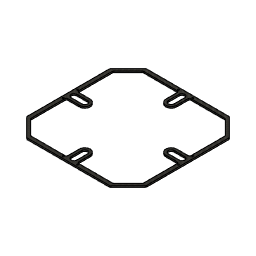
CarbonFiberBoardDown (Autodesk Fusion 360 design; units mm, degrees)
Autodesk Fusion 360 part; units mm, degrees
sketch "草图1" plane through (0, 0, 0) normal (0, 0, 1) x (1, 0, 0)
  line L0 (7.5, 60) -> (7.5, 75)
  circle A0 centre (-42.5, 42.5) radius 32.5 construction
  arc A1 (-7.5, 60) -> (7.5, 60) centre (0, 60) ccw
  circle A2 centre (42.5, 42.5) radius 32.5 construction
  circle A3 centre (-10, 80) radius 1.05
  line L1 (-7.5, 75) -> (-7.5, 60)
  line L2 (57.8614, 83) -> (0, 83)
  line L3 (0, 60) -> (0, 75) construction
  circle A4 centre (10, 80) radius 1.05
  circle A5 centre (42.5, -42.5) radius 32.5 construction
  circle A6 centre (-42.5, -42.5) radius 32.5 construction
  arc A7 (7.5, 75) -> (-7.5, 75) centre (0, 75) ccw construction
  line L4 (7.5, 75) -> (7.5, 78)
  line L5 (7.5, 78) -> (57.2046, 78)
  line L6 (0, 0) -> (89.0494, 89.0494) construction
  line L7 (57.2046, 78) -> (67.6023, 67.6023)
  line L8 (57.8614, 83) -> (70.4307, 70.4307)
  line L9 (-57.8614, 83) -> (0, 83)
  line L10 (-57.8614, 83) -> (-70.4307, 70.4307)
  line L11 (-57.2046, 78) -> (-67.6023, 67.6023)
  line L12 (-7.5, 78) -> (-57.2046, 78)
  line L13 (-7.5, 75) -> (-7.5, 78)
  line L14 (-4, 75) -> (-4, 60)
  arc A8 (-4, 60) -> (4, 60) centre (0, 60) ccw
  line L15 (4, 60) -> (4, 75)
  arc A9 (4, 75) -> (-4, 75) centre (0, 75) ccw
  line L16 (0, 75) -> (0, 60) construction
  line L17 (-83, -57.8614) -> (-70.4307, -70.4307)
  line L18 (-83, -57.8614) -> (-83, 0)
  line L19 (-83, 57.8614) -> (-83, 0)
  line L20 (-83, 57.8614) -> (-70.4307, 70.4307)
  line L21 (-78, 57.2046) -> (-67.6023, 67.6023)
  line L22 (-78, 7.5) -> (-78, 57.2046)
  line L23 (-75, 7.5) -> (-78, 7.5)
  line L24 (-60, 7.5) -> (-75, 7.5)
  arc A10 (-60, -7.5) -> (-60, 7.5) centre (-60, 0) ccw
  line L25 (-75, -7.5) -> (-60, -7.5)
  line L26 (-75, -7.5) -> (-78, -7.5)
  line L27 (-78, -7.5) -> (-78, -57.2046)
  line L28 (-78, -57.2046) -> (-67.6023, -67.6023)
  line L29 (-75, -4) -> (-60, -4)
  arc A11 (-75, 4) -> (-75, -4) centre (-75, 0) ccw
  line L30 (-60, 4) -> (-75, 4)
  arc A12 (-60, -4) -> (-60, 4) centre (-60, 0) ccw
  circle A13 centre (-80, -10) radius 1.05
  circle A14 centre (-80, 10) radius 1.05
  line L31 (57.8614, -83) -> (70.4307, -70.4307)
  line L32 (57.8614, -83) -> (0, -83)
  line L33 (-57.8614, -83) -> (0, -83)
  line L34 (-57.8614, -83) -> (-70.4307, -70.4307)
  line L35 (-57.2046, -78) -> (-67.6023, -67.6023)
  line L36 (-7.5, -78) -> (-57.2046, -78)
  line L37 (-7.5, -75) -> (-7.5, -78)
  line L38 (-7.5, -60) -> (-7.5, -75)
  arc A15 (7.5, -60) -> (-7.5, -60) centre (0, -60) ccw
  line L39 (7.5, -75) -> (7.5, -60)
  line L40 (7.5, -75) -> (7.5, -78)
  line L41 (7.5, -78) -> (57.2046, -78)
  line L42 (57.2046, -78) -> (67.6023, -67.6023)
  line L43 (4, -75) -> (4, -60)
  arc A16 (-4, -75) -> (4, -75) centre (0, -75) ccw
  line L44 (-4, -60) -> (-4, -75)
  arc A17 (4, -60) -> (-4, -60) centre (0, -60) ccw
  circle A18 centre (10, -80) radius 1.05
  circle A19 centre (-10, -80) radius 1.05
  line L45 (83, 57.8614) -> (70.4307, 70.4307)
  line L46 (83, 57.8614) -> (83, 0)
  line L47 (83, -57.8614) -> (83, 0)
  line L48 (83, -57.8614) -> (70.4307, -70.4307)
  line L49 (78, -57.2046) -> (67.6023, -67.6023)
  line L50 (78, -7.5) -> (78, -57.2046)
  line L51 (75, -7.5) -> (78, -7.5)
  line L52 (60, -7.5) -> (75, -7.5)
  arc A20 (60, 7.5) -> (60, -7.5) centre (60, 0) ccw
  line L53 (75, 7.5) -> (60, 7.5)
  line L54 (75, 7.5) -> (78, 7.5)
  line L55 (78, 7.5) -> (78, 57.2046)
  line L56 (78, 57.2046) -> (67.6023, 67.6023)
  line L57 (75, 4) -> (60, 4)
  arc A21 (75, -4) -> (75, 4) centre (75, 0) ccw
  line L58 (60, -4) -> (75, -4)
  arc A22 (60, 4) -> (60, -4) centre (60, 0) ccw
  circle A23 centre (80, 10) radius 1.05
  circle A24 centre (80, -10) radius 1.05
  dimension "d3" = 65
  dimension "d4" = 65
  dimension "d5" = 65
  dimension "d6" = 65
  dimension "d7" = 15
  dimension "d8" = 15
  dimension "d10" = 2.1
  dimension "d11" = 5
  dimension "d12" = 10
  dimension "d15" = 3
  dimension "d16" = 2
  dimension "d17" = 60
  dimension "d18" = 35.5
  dimension "d19" = 4
  dimension "d20" = 8
  dimension "d22" = 360
  constraint tangent L0 A7
  constraint tangent L1 A7
  constraint parallel L0 L1
  constraint tangent A1 L1
  constraint tangent L0 A1
  constraint vertical L3
  constraint horizontal L2
  constraint symmetric A3 L3 A4
  constraint tangent A7 L4
  constraint perpendicular L0 L5
  constraint coincident L6.start origin
  constraint coincident A2.centre L6
  constraint vertical L2.end L3.end
  constraint coincident L6 L7.end
  constraint perpendicular L6 L7
  constraint vertical L6.start A1.centre
  constraint coincident L6 L8.end
  constraint perpendicular L6 L8
  constraint symmetric L2.end L3 L9.end
  constraint symmetric L2.start L3 L9.start
  constraint symmetric L0.end L3 L1.start
  constraint symmetric L3 L4.end L12.start
  constraint symmetric L3 L5.end L11.start
  constraint symmetric L3 L7.end L11.end
  constraint symmetric L3 L8.end L10.end
  constraint tangent L14 A8
  constraint tangent A8 L15
  constraint parallel L14 L15
  constraint tangent L15 A9
  constraint tangent L14 A9
  constraint coincident A1.centre L3.start
  constraint perpendicular L9 L16
  constraint coincident L3.end A7.centre
  measures "d3" diameter of A5
  measures "d4" diameter of A6
  measures "d5" diameter of A0
  measures "d6" diameter of A2
  measures "d7" distance of L0 L1
  measures "d8" distance of A1.centre L3.end
  measures "d10" diameter of A4
  measures "d11" vertical distance of L3.end A4.centre
  measures "d12" horizontal distance of L3.end A4.centre
  measures "d15" distance of A4.centre L2
  measures "d16" distance of A4.centre L5
  measures "d17" distance of L6.start A1.centre
  measures "d18" distance of A2.centre L7.end
  measures "d19" distance of L7 L8
  measures "d20" distance of L14 L15
extrude "拉伸1" add sketch "草图1" along normal blind 2
fillet "圆角1" radius 2 16 edges at (-57.2046, 78, 1) (57.2046, 78, 1) (78, 57.2046, 1) (-7.5, 78, 1) (7.5, 78, 1) (78, 7.5, 1) (78, -7.5, 1) (78, -57.2046, 1) (57.2046, -78, 1) (7.5, -78, 1) (-7.5, -78, 1) (-57.2046, -78, 1) (-78, -57.2046, 1) (-78, -7.5, 1) (-78, 7.5, 1) (-78, 57.2046, 1)
fillet "圆角2" radius 2 8 edges at (83, -57.8614, 1) (57.8614, -83, 1) (-57.8614, -83, 1) (-83, -57.8614, 1) (-83, 57.8614, 1) (-57.8614, 83, 1) (57.8614, 83, 1) (83, 57.8614, 1)
